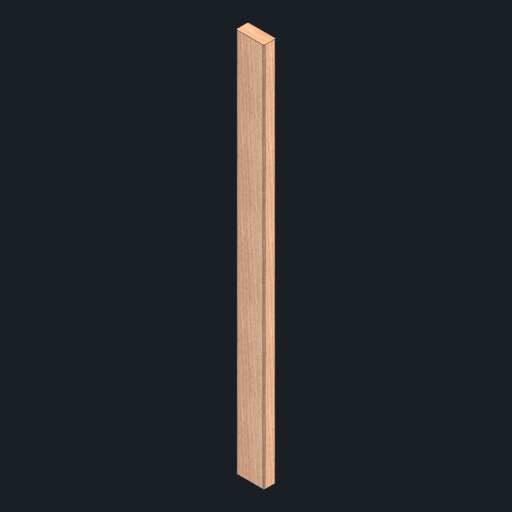
# Autodesk Inventor part: Horizontal Beam 4ft
Saved by Autodesk Inventor 2024.2 (Build 282272000, 272)
## iProperties
Created: 2025-06-28
Part Number: Horizontal Beam 4ft
Material: Wood (Birch)
Document SubType Name: Modeling
Designer: Bryan
Density: 0.55 g/cm^3
Appearance: Birch - Natural Polished
Author: Bryan
Autodesk Inventor part; units mm, degrees
ref_plane "YZ Plane" through (0, 0, 0) normal (1, 0, 0) x (0, 1, 0)
ref_plane "XZ Plane" through (0, 0, 0) normal (0, 1, 0) x (-1, 0, 0)
ref_plane "XY Plane" through (0, 0, 0) normal (0, 0, 1) x (1, 0, 0)
sketch "Sketch1" plane through (0, 0, 0) normal (0, 1, 0) x (-1, 0, 0)
  line L0 (3.175, 0) -> (85.725, 0)
  line L1 (88.9, -3.175) -> (88.9, -34.925)
  line L2 (85.725, -38.1) -> (3.175, -38.1)
  line L3 (0, -34.925) -> (0, -3.175)
  arc A0 (88.9, -3.175) -> (85.725, 0) centre (85.725, -3.175) ccw
  arc A1 (85.725, -38.1) -> (88.9, -34.925) centre (85.725, -34.925) ccw
  arc A2 (0, -34.925) -> (3.175, -38.1) centre (3.175, -34.925) ccw
  arc A3 (3.175, 0) -> (0, -3.175) centre (3.175, -3.175) ccw
  point P0 (0, 0)
  point P1 (88.9, -38.1)
  point P2 (88.9, 0)
  point P3 (0, -38.1)
  dimension "d0" = 88.9
  dimension "d1" = 38.1
  dimension "d2" = 3.175
  constraints: 8 end point, 8 point on circle, 8 point on line, 8 tangent, 4 centre point, 3 equal radius, 2 parallel, 1 horizontal, 1 perpendicular
  measures "d0" distance of point (88.9, -38.1) point (0, -38.1)
  measures "d1" distance of point (88.9, 0) point (88.9, -38.1)
  measures "d2" radius of A0
extrude "Extrusion1" add sketch "Sketch1" along normal blind 1219.2
body "Solid1"
